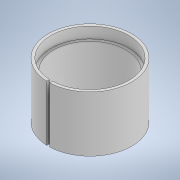
# Autodesk Inventor part: zig64
Saved by Autodesk Inventor 2022 (Build 260153000, 153)
## iProperties
Created: 2022-03-02
Part Number: zig64
Material: Generic
Document SubType Name: Modeling
Designer: Yazawa
Density: 1 g/cm^3
Appearance: Default
Author: Yazawa
Autodesk Inventor part; units mm, degrees
ref_plane "YZ Plane" through (0, 0, 0) normal (1, 0, 0) x (0, 1, 0)
ref_plane "XZ Plane" through (0, 0, 0) normal (0, 1, 0) x (-1, 0, 0)
ref_plane "XY Plane" through (0, 0, 0) normal (0, 0, 1) x (1, 0, 0)
sketch "スケッチ1" plane through (0, 0, 0) normal (0, 1, 0) x (-1, 0, 0)
  circle A0 centre (0, 0) radius 7
  circle A1 centre (0, 0) radius 7.5
  dimension "d0" = 14
  dimension "d1" = 15
  constraints: 2 centre point, 2 coincident
  measures "d0" diameter of A0
  measures "d1" diameter of A1
extrude "押し出し1" add sketch "スケッチ1" along normal blind 10
sketch "スケッチ2" plane through (0, 0, 0) normal (0, -1, 0) x (1, 0, 0)
  circle A0 centre (0, 0) radius 6.5
  circle A1 centre (0, 0) radius 7 projected
  dimension "d4" = 13
  constraints: 1 centre point, 1 coincident
  measures "d4" diameter of A0
extrude "押し出し2" add sketch "スケッチ2" against normal blind 8
sketch "スケッチ3" plane through (0, 10, 0) normal (0, 1, 0) x (1, 0, 0)
  line L0 (0.25, -1.8599) -> (0.25, -7.9917)
  line L1 (0.25, -7.9917) -> (-0.25, -7.9917)
  line L2 (-0.25, -7.9917) -> (-0.25, -1.8599)
  line L3 (-0.25, -1.8599) -> (0, -1.8599)
  line L4 (0, -1.8599) -> (0.25, -1.8599)
  point P0 (0, 0)
  dimension "d7" = 0.5
  constraints: 10 end point, 2 equal length, 1 collinear, 1 horizontal, 1 vertical, 1 vertical alignment
  measures "d7" distance of L0.end L1.end
extrude "押し出し3" cut sketch "スケッチ3" against normal through all
